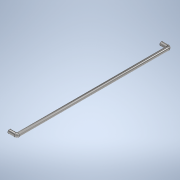
# Autodesk Inventor part: Styrepind
Saved by Autodesk Inventor 2020.4 (Build 244396000, 396)
## iProperties
Created: 2021-05-01
Part Number: Styrepind
Material: Steel
Document SubType Name: Modeling
Designer: armin
Density: 7.85 g/cm^3
Appearance: Knurled 45
Author: armin
Autodesk Inventor part; units mm, degrees
ref_plane "YZ Plane" through (0, 0, 0) normal (1, 0, 0) x (0, 1, 0)
ref_plane "XZ Plane" through (0, 0, 0) normal (0, 1, 0) x (-1, 0, 0)
ref_plane "XY Plane" through (0, 0, 0) normal (0, 0, 1) x (1, 0, 0)
sketch "Sketch1" plane through (0, 0, 0) normal (1, 0, 0) x (0, 1, 0)
  circle A0 centre (0, 0) radius 1
  dimension "d0" = 2
  constraints: 1 centre point, 1 coincident
  measures "d0" diameter of A0
sketch "Sketch2" plane through (0, 0, 0) normal (0, 1, 0) x (-1, 0, 0)
  line L0 (0, 0) -> (-3.5, 0)
  line L1 (-4, -0.5) -> (-4, -84.5)
  line L2 (-3.5, -85) -> (0, -85)
  arc A0 (-3.5, 0) -> (-4, -0.5) centre (-3.5, -0.5) ccw
  arc A1 (-4, -84.5) -> (-3.5, -85) centre (-3.5, -84.5) ccw
  point P0 (-4, 0)
  point P1 (-4, -85)
  dimension "d1" = 4
  dimension "d2" = 85
  dimension "d3" = 0.5
  constraints: 6 end point, 4 point on circle, 4 point on line, 4 tangent, 2 centre point, 2 perpendicular, 1 equal radius, 1 horizontal
  measures "d1" distance of L0.start point (-4, 0)
  measures "d2" distance of point (-4, 0) point (-4, -85)
  measures "d3" radius of A0
sweep "Sweep1" add profiles "Sketch1" path "Sketch2"
body "Solid1"
